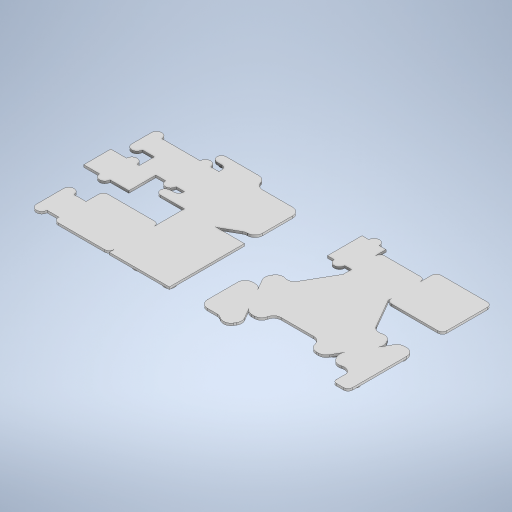
# Autodesk Inventor part: CORE_set_outline
Saved by Autodesk Inventor 2024.1 (Build 281209000, 209)
## iProperties
Created: 2025-04-12
Part Number: CORE_set_outline
Material: 一般
Document SubType Name: Modeling
Designer: hibik
Density: 1 g/cm^3
Appearance: 既定
Author: hibik
Autodesk Inventor part; units mm, degrees
ref_plane "YZ Plane" through (0, 0, 0) normal (1, 0, 0) x (0, 1, 0)
ref_plane "XZ Plane" through (0, 0, 0) normal (0, 1, 0) x (-1, 0, 0)
ref_plane "XY Plane" through (0, 0, 0) normal (0, 0, 1) x (1, 0, 0)
sketch "スケッチ8" plane through (0, 0, 0) normal (0, 1, 0) x (-1, 0, 0)
  line L0 (15, -121.1) -> (15, -99.7075) projected
  arc A0 (15.25, -99.213) -> (15, -99.7075) centre (19.5802, -101.713) ccw projected
  line L1 (15.25, -99.213) -> (26.142, -80.3476) projected
  arc A1 (32.0798, -78.1131) -> (26.142, -80.3476) centre (30.4721, -82.8476) ccw projected
  arc A2 (32.0798, -78.1131) -> (38.0175, -75.8786) centre (33.6874, -73.3786) ccw projected
  line L2 (38.0175, -75.8786) -> (38.7859, -74.5477) projected
  arc A3 (38.7859, -74.5477) -> (38.7859, -69.5477) centre (34.4558, -72.0477) ccw projected
  line L3 (38.7859, -69.5477) -> (26.6628, -48.55) projected
  arc A4 (26.6628, -48.55) -> (22.3327, -46.05) centre (22.3327, -51.05) ccw projected
  line L4 (22.3327, -46.05) -> (20.604, -46.05) projected
  arc A5 (20.604, -46.05) -> (15.7, -50.075) centre (20.604, -51.05) ccw projected
  arc A6 (10.796, -54.1) -> (15.7, -50.075) centre (10.796, -49.1) ccw projected
  line L5 (10.796, -54.1) -> (-10.988, -54.1) projected
  arc A7 (-15.892, -50.075) -> (-10.988, -54.1) centre (-10.988, -49.1) ccw projected
  arc A8 (-15.892, -50.075) -> (-20.796, -46.05) centre (-20.796, -51.05) ccw projected
  line L6 (-20.796, -46.05) -> (-22.3327, -46.05) projected
  arc A9 (-22.3327, -46.05) -> (-26.6628, -48.55) centre (-22.3327, -51.05) ccw projected
  line L7 (-26.6628, -48.55) -> (-38.7859, -69.5477) projected
  arc A10 (-38.7859, -69.5477) -> (-38.7859, -74.5477) centre (-34.4558, -72.0477) ccw projected
  line L8 (-38.7859, -74.5477) -> (-37.9215, -76.0448) projected
  arc A11 (-37.9215, -76.0448) -> (-31.9838, -78.2793) centre (-33.5914, -73.5448) ccw projected
  arc A12 (-26.046, -80.5138) -> (-31.9838, -78.2793) centre (-30.3761, -83.0138) ccw projected
  line L9 (-26.046, -80.5138) -> (-15.154, -99.3793) projected
  arc A13 (-15, -99.6675) -> (-15.154, -99.3793) centre (-19.4842, -101.8793) ccw projected
  line L10 (-15, -99.6675) -> (-15, -121.1) projected
  arc A14 (-15, -121.1) -> (-12, -124.1) centre (-12, -121.1) ccw projected
  line L11 (-12, -124.1) -> (12, -124.1) projected
  arc A15 (12, -124.1) -> (15, -121.1) centre (12, -121.1) ccw projected
  arc A16 (-43.4038, -36.5236) -> (-45.4038, -34.5236) centre (-45.4038, -36.5236) ccw projected
  line L12 (-45.4038, -34.5236) -> (-50.4038, -34.5236) projected
  arc A17 (-50.4038, -34.5236) -> (-53.4038, -37.5236) centre (-50.4038, -37.5236) ccw projected
  line L13 (-53.4038, -37.5236) -> (-53.4038, -73.5448) projected
  arc A18 (-53.4038, -73.5448) -> (-48.4038, -78.5448) centre (-48.4038, -73.5448) ccw projected
  line L14 (-48.4038, -78.5448) -> (-46.8671, -78.5448) projected
  arc A19 (-46.8671, -78.5448) -> (-42.537, -76.0448) centre (-46.8671, -73.5448) ccw projected
  line L15 (-42.537, -76.0448) -> (-30.4139, -55.0471) projected
  arc A20 (-30.4139, -55.0471) -> (-30.4139, -50.0471) centre (-34.7441, -52.5471) ccw projected
  line L16 (-30.4139, -50.0471) -> (-31.2783, -48.55) projected
  arc A21 (-31.2783, -48.55) -> (-37.2161, -46.3155) centre (-35.6084, -51.05) ccw projected
  arc A22 (-43.1538, -44.081) -> (-37.2161, -46.3155) centre (-38.8237, -41.581) ccw projected
  line L17 (-43.1538, -44.081) -> (-43.4038, -43.6479) projected
  line L18 (-43.4038, -43.6479) -> (-43.4038, -36.5236) projected
  arc A23 (-49, -98.6929) -> (-52, -101.6929) centre (-49, -101.6929) ccw projected
  line L19 (-52, -101.6929) -> (-52, -128.6929) projected
  arc A24 (-52, -128.6929) -> (-49, -131.6929) centre (-49, -128.6929) ccw projected
  line L20 (-49, -131.6929) -> (-18, -131.6929) projected
  arc A25 (-18, -131.6929) -> (-15, -128.6929) centre (-18, -128.6929) ccw projected
  line L21 (-15, -128.6929) -> (-15, -101.6929) projected
  arc A26 (-15, -101.6929) -> (-18, -98.6929) centre (-18, -101.6929) ccw projected
  line L22 (-18, -98.6929) -> (-49, -98.6929) projected
  line L23 (26.5, -128.1929) -> (31, -128.1929) projected
  line L24 (31, -128.1929) -> (31, -105.1929) projected
  line L25 (31, -105.1929) -> (26.5, -105.1929) projected
  arc A27 (26.5, -105.1929) -> (19.5, -105.1929) centre (23, -105.1929) ccw projected
  line L26 (19.5, -105.1929) -> (15, -105.1929) projected
  line L27 (15, -105.1929) -> (15, -128.1929) projected
  line L28 (15, -128.1929) -> (19.5, -128.1929) projected
  arc A28 (19.5, -128.1929) -> (26.5, -128.1929) centre (23, -128.1929) ccw projected
  arc A29 (45.5962, -39.8878) -> (40.5962, -34.8878) centre (40.5962, -39.8878) ccw projected
  line L29 (40.5962, -34.8878) -> (34.1859, -34.8878) projected
  arc A30 (31.6859, -34.2179) -> (34.1859, -34.8878) centre (34.1859, -29.8878) ccw projected
  line L30 (31.6859, -34.2179) -> (30.2047, -33.3628) projected
  arc A31 (30.2047, -33.3628) -> (23.3746, -35.1929) centre (27.7047, -37.6929) ccw projected
  line L31 (23.3746, -35.1929) -> (22.6062, -36.5238) projected
  arc A32 (22.6062, -36.5238) -> (22.6062, -41.5238) centre (26.9364, -39.0238) ccw projected
  line L32 (22.6062, -41.5238) -> (34.7293, -62.5215) projected
  arc A33 (34.7293, -62.5215) -> (39.0594, -65.0215) centre (39.0594, -60.0215) ccw projected
  line L33 (39.0594, -65.0215) -> (40.5962, -65.0215) projected
  arc A34 (40.5962, -65.0215) -> (45.5962, -60.0215) centre (40.5962, -60.0215) ccw projected
  line L34 (45.5962, -60.0215) -> (45.5962, -39.8878) projected
  arc A35 (70.5962, -91.5196) -> (65.5962, -96.5196) centre (70.5962, -96.5196) ccw projected
  line L35 (65.5962, -96.5196) -> (65.5962, -116.5196) projected
  arc A36 (65.5962, -116.5196) -> (70.5962, -121.5196) centre (70.5962, -116.5196) ccw projected
  line L36 (70.5962, -121.5196) -> (90.5124, -121.5196) projected
  arc A37 (95.2815, -125.0175) -> (90.5124, -121.5196) centre (90.5124, -126.5196) ccw projected
  arc A38 (95.2815, -125.0175) -> (100.0506, -128.5155) centre (100.0506, -123.5155) ccw projected
  line L37 (100.0506, -128.5155) -> (121.8354, -128.5155) projected
  arc A39 (121.8354, -128.5155) -> (123.6192, -123.1035) centre (121.8354, -125.5155) ccw projected
  arc A40 (123.6192, -123.1035) -> (122.0183, -122.3155) centre (120.6462, -127.1236) ccw projected
  line L38 (122.0183, -122.3155) -> (118.5962, -122.3155) projected
  arc A41 (115.5962, -119.3155) -> (118.5962, -122.3155) centre (118.5962, -119.3155) ccw projected
  line L39 (115.5962, -119.3155) -> (115.5962, -93.7236) projected
  arc A42 (118.5962, -90.7236) -> (115.5962, -93.7236) centre (118.5962, -93.7236) ccw projected
  line L40 (118.5962, -90.7236) -> (121.224, -90.7236) projected
  arc A43 (121.6212, -90.6276) -> (121.224, -90.7236) centre (122.5962, -95.5316) ccw projected
  arc A44 (121.6212, -90.6276) -> (122.8256, -90.2236) centre (120.6462, -85.7236) ccw projected
  arc A45 (122.8256, -90.2236) -> (121.5179, -84.5236) centre (121.5179, -87.5236) ccw projected
  line L41 (121.5179, -84.5236) -> (84.9713, -84.5236) projected
  arc A46 (84.9713, -84.5236) -> (83.4713, -84.9255) centre (84.9713, -87.5236) ccw projected
  line L42 (83.4713, -84.9255) -> (73.2103, -90.8497) projected
  arc A47 (70.7103, -91.5196) -> (73.2103, -90.8497) centre (70.7103, -86.5196) ccw projected
  line L43 (70.7103, -91.5196) -> (70.5962, -91.5196) projected
  line L44 (121.0962, -94.5155) -> (115.5962, -94.5155) projected
  line L45 (115.5962, -94.5155) -> (115.5962, -117.5155) projected
  line L46 (115.5962, -117.5155) -> (121.0962, -117.5155) projected
  arc A48 (121.0962, -117.5155) -> (128.0962, -117.5155) centre (124.5962, -117.5155) ccw projected
  line L47 (128.0962, -117.5155) -> (145.5962, -117.5155) projected
  line L48 (145.5962, -117.5155) -> (145.5962, -94.5155) projected
  line L49 (145.5962, -94.5155) -> (128.0962, -94.5155) projected
  arc A49 (128.0962, -94.5155) -> (121.0962, -94.5155) centre (124.5962, -94.5155) ccw projected
  line L50 (153.5962, -104.5155) -> (145.5962, -104.5155) projected
  line L51 (145.5962, -104.5155) -> (145.5962, -117.5155) projected
  line L52 (145.5962, -117.5155) -> (153.5962, -117.5155) projected
  arc A50 (153.5962, -117.5155) -> (160.5962, -117.5155) centre (157.0962, -117.5155) ccw projected
  line L53 (160.5962, -117.5155) -> (160.5962, -104.5155) projected
  arc A51 (160.5962, -104.5155) -> (153.5962, -104.5155) centre (157.0962, -104.5155) ccw projected
  line L54 (147.0962, -76.5155) -> (134.5962, -76.5155) projected
  line L55 (134.5962, -76.5155) -> (134.5962, -94.5155) projected
  line L56 (134.5962, -94.5155) -> (147.0962, -94.5155) projected
  arc A52 (147.0962, -94.5155) -> (154.0962, -94.5155) centre (150.5962, -94.5155) ccw projected
  line L57 (154.0962, -94.5155) -> (164.5962, -94.5155) projected
  line L58 (164.5962, -94.5155) -> (164.5962, -76.5155) projected
  line L59 (164.5962, -76.5155) -> (154.0962, -76.5155) projected
  arc A53 (154.0962, -76.5155) -> (147.0962, -76.5155) centre (150.5962, -76.5155) ccw projected
  line L60 (65.5962, -84.5236) -> (105.5962, -84.5236) projected
  line L61 (105.5962, -84.5236) -> (105.5962, -54.5236) projected
  line L62 (105.5962, -54.5236) -> (65.5962, -54.5236) projected
  line L63 (65.5962, -54.5236) -> (65.5962, -84.5236) projected
  line L64 (65.5962, -54.5236) -> (105.5962, -54.5236) projected
  line L65 (105.5962, -54.5236) -> (105.5962, -34.5236) projected
  line L66 (105.5962, -34.5236) -> (65.5962, -34.5236) projected
  line L67 (65.5962, -34.5236) -> (65.5962, -54.5236) projected
  arc A54 (108.5962, -34.5236) -> (105.5962, -37.5236) centre (108.5962, -37.5236) ccw projected
  line L68 (105.5962, -37.5236) -> (105.5962, -64.5236) projected
  arc A55 (105.5962, -64.5236) -> (108.5962, -67.5236) centre (108.5962, -64.5236) ccw projected
  line L69 (108.5962, -67.5236) -> (139.5962, -67.5236) projected
  arc A56 (139.5962, -67.5236) -> (142.5962, -64.5236) centre (139.5962, -64.5236) ccw projected
  line L70 (142.5962, -64.5236) -> (142.5962, -37.5236) projected
  arc A57 (142.5962, -37.5236) -> (139.5962, -34.5236) centre (139.5962, -37.5236) ccw projected
  line L71 (139.5962, -34.5236) -> (108.5962, -34.5236) projected
  line L72 (157.5962, -56.0236) -> (157.5962, -38.0236) projected
  arc A58 (157.5962, -38.0236) -> (150.5962, -38.0236) centre (154.0962, -38.0236) ccw projected
  line L73 (150.5962, -38.0236) -> (142.5962, -38.0236) projected
  line L74 (142.5962, -38.0236) -> (142.5962, -56.0236) projected
  line L75 (142.5962, -56.0236) -> (150.5962, -56.0236) projected
  arc A59 (150.5962, -56.0236) -> (157.5962, -56.0236) centre (154.0962, -56.0236) ccw projected
  point P0 (0, 0)
extrude "押し出し6" add sketch "スケッチ8" along normal blind 1.5
sketch "スケッチ9" plane through (0, 1.5, 0) normal (0, 1, 0) x (1, 0, 0)
  line L0 (-22.6062, 41.5238) -> (-26.6628, 48.55) projected
  arc A0 (-26.6628, 48.55) -> (-22.3327, 46.05) centre (-22.3327, 51.05) ccw projected
  line L1 (-22.3327, 46.05) -> (-20.604, 46.05) projected
  arc A1 (-20.604, 46.05) -> (-15.7, 50.075) centre (-20.604, 51.05) ccw projected
  arc A2 (-10.796, 54.1) -> (-15.7, 50.075) centre (-10.796, 49.1) ccw projected
  line L2 (-10.796, 54.1) -> (10.988, 54.1) projected
  arc A3 (15.892, 50.075) -> (10.988, 54.1) centre (10.988, 49.1) ccw projected
  arc A4 (15.892, 50.075) -> (20.796, 46.05) centre (20.796, 51.05) ccw projected
  line L3 (20.796, 46.05) -> (22.3327, 46.05) projected
  arc A5 (22.3327, 46.05) -> (26.6628, 48.55) centre (22.3327, 51.05) ccw projected
  line L4 (26.6628, 48.55) -> (30.4139, 55.0471) projected
  arc A6 (30.4139, 55.0471) -> (30.4139, 50.0471) centre (34.7441, 52.5471) ccw projected
  line L5 (30.4139, 50.0471) -> (31.2783, 48.55) projected
  arc A7 (31.2783, 48.55) -> (37.2161, 46.3155) centre (35.6084, 51.05) ccw projected
  arc A8 (43.1538, 44.081) -> (37.2161, 46.3155) centre (38.8237, 41.581) ccw projected
  line L6 (43.1538, 44.081) -> (43.4038, 43.6479) projected
  line L7 (43.4038, 43.6479) -> (43.4038, 36.5236) projected
  arc A9 (43.4038, 36.5236) -> (45.4038, 34.5236) centre (45.4038, 36.5236) ccw projected
  line L8 (45.4038, 34.5236) -> (50.4038, 34.5236) projected
  arc A10 (50.4038, 34.5236) -> (53.4038, 37.5236) centre (50.4038, 37.5236) ccw projected
  line L9 (53.4038, 37.5236) -> (53.4038, 73.5448) projected
  arc A11 (53.4038, 73.5448) -> (48.4038, 78.5448) centre (48.4038, 73.5448) ccw projected
  line L10 (48.4038, 78.5448) -> (46.8671, 78.5448) projected
  arc A12 (46.8671, 78.5448) -> (42.537, 76.0448) centre (46.8671, 73.5448) ccw projected
  line L11 (42.537, 76.0448) -> (38.7859, 69.5477) projected
  arc A13 (38.7859, 69.5477) -> (38.7859, 74.5477) centre (34.4558, 72.0477) ccw projected
  line L12 (38.7859, 74.5477) -> (37.9215, 76.0448) projected
  arc A14 (37.9215, 76.0448) -> (31.9838, 78.2793) centre (33.5914, 73.5448) ccw projected
  arc A15 (26.046, 80.5138) -> (31.9838, 78.2793) centre (30.3761, 83.0138) ccw projected
  line L13 (26.046, 80.5138) -> (15.154, 99.3793) projected
  arc A16 (15, 99.6675) -> (15.154, 99.3793) centre (19.4842, 101.8793) ccw projected
  line L14 (15, 99.6675) -> (15, 101.6929) projected
  arc A17 (15, 101.6929) -> (18, 98.6929) centre (18, 101.6929) ccw projected
  line L15 (18, 98.6929) -> (49, 98.6929) projected
  arc A18 (49, 98.6929) -> (52, 101.6929) centre (49, 101.6929) ccw projected
  line L16 (52, 101.6929) -> (52, 128.6929) projected
  arc A19 (52, 128.6929) -> (49, 131.6929) centre (49, 128.6929) ccw projected
  line L17 (49, 131.6929) -> (18, 131.6929) projected
  arc A20 (18, 131.6929) -> (15, 128.6929) centre (18, 128.6929) ccw projected
  line L18 (15, 128.6929) -> (15, 121.1) projected
  arc A21 (15, 121.1) -> (12, 124.1) centre (12, 121.1) ccw projected
  line L19 (12, 124.1) -> (-12, 124.1) projected
  arc A22 (-12, 124.1) -> (-15, 121.1) centre (-12, 121.1) ccw projected
  line L20 (-15, 121.1) -> (-15, 128.1929) projected
  line L21 (-15, 128.1929) -> (-19.5, 128.1929) projected
  arc A23 (-19.5, 128.1929) -> (-26.5, 128.1929) centre (-23, 128.1929) ccw projected
  line L22 (-26.5, 128.1929) -> (-31, 128.1929) projected
  line L23 (-31, 128.1929) -> (-31, 105.1929) projected
  line L24 (-31, 105.1929) -> (-26.5, 105.1929) projected
  arc A24 (-26.5, 105.1929) -> (-19.5, 105.1929) centre (-23, 105.1929) ccw projected
  line L25 (-19.5, 105.1929) -> (-15, 105.1929) projected
  line L26 (-15, 105.1929) -> (-15, 99.7075) projected
  arc A25 (-15.25, 99.213) -> (-15, 99.7075) centre (-19.5802, 101.713) ccw projected
  line L27 (-15.25, 99.213) -> (-26.142, 80.3476) projected
  arc A26 (-32.0798, 78.1131) -> (-26.142, 80.3476) centre (-30.4721, 82.8476) ccw projected
  arc A27 (-32.0798, 78.1131) -> (-38.0175, 75.8786) centre (-33.6874, 73.3786) ccw projected
  line L28 (-38.0175, 75.8786) -> (-38.7859, 74.5477) projected
  arc A28 (-38.7859, 74.5477) -> (-38.7859, 69.5477) centre (-34.4558, 72.0477) ccw projected
  line L29 (-38.7859, 69.5477) -> (-34.7293, 62.5215) projected
  arc A29 (-34.7293, 62.5215) -> (-39.0594, 65.0215) centre (-39.0594, 60.0215) ccw projected
  line L30 (-39.0594, 65.0215) -> (-40.5962, 65.0215) projected
  arc A30 (-40.5962, 65.0215) -> (-45.5962, 60.0215) centre (-40.5962, 60.0215) ccw projected
  line L31 (-45.5962, 60.0215) -> (-45.5962, 39.8878) projected
  arc A31 (-45.5962, 39.8878) -> (-40.5962, 34.8878) centre (-40.5962, 39.8878) ccw projected
  line L32 (-40.5962, 34.8878) -> (-34.1859, 34.8878) projected
  arc A32 (-31.6859, 34.2179) -> (-34.1859, 34.8878) centre (-34.1859, 29.8878) ccw projected
  line L33 (-31.6859, 34.2179) -> (-30.2047, 33.3628) projected
  arc A33 (-30.2047, 33.3628) -> (-23.3746, 35.1929) centre (-27.7047, 37.6929) ccw projected
  line L34 (-23.3746, 35.1929) -> (-22.6062, 36.5238) projected
  arc A34 (-22.6062, 36.5238) -> (-22.6062, 41.5238) centre (-26.9364, 39.0238) ccw projected
  line L35 (-65.5962, 84.5236) -> (-84.9713, 84.5236) projected
  arc A35 (-84.9713, 84.5236) -> (-83.4713, 84.9255) centre (-84.9713, 87.5236) ccw projected
  line L36 (-83.4713, 84.9255) -> (-73.2103, 90.8497) projected
  arc A36 (-70.7103, 91.5196) -> (-73.2103, 90.8497) centre (-70.7103, 86.5196) ccw projected
  line L37 (-70.7103, 91.5196) -> (-70.5962, 91.5196) projected
  arc A37 (-70.5962, 91.5196) -> (-65.5962, 96.5196) centre (-70.5962, 96.5196) ccw projected
  line L38 (-65.5962, 96.5196) -> (-65.5962, 116.5196) projected
  arc A38 (-65.5962, 116.5196) -> (-70.5962, 121.5196) centre (-70.5962, 116.5196) ccw projected
  line L39 (-70.5962, 121.5196) -> (-90.5124, 121.5196) projected
  arc A39 (-95.2815, 125.0175) -> (-90.5124, 121.5196) centre (-90.5124, 126.5196) ccw projected
  arc A40 (-95.2815, 125.0175) -> (-100.0506, 128.5155) centre (-100.0506, 123.5155) ccw projected
  line L40 (-100.0506, 128.5155) -> (-121.8354, 128.5155) projected
  arc A41 (-121.8354, 128.5155) -> (-123.6192, 123.1035) centre (-121.8354, 125.5155) ccw projected
  arc A42 (-123.6192, 123.1035) -> (-122.0183, 122.3155) centre (-120.6462, 127.1236) ccw projected
  line L41 (-122.0183, 122.3155) -> (-118.5962, 122.3155) projected
  arc A43 (-115.5962, 119.3155) -> (-118.5962, 122.3155) centre (-118.5962, 119.3155) ccw projected
  line L42 (-115.5962, 119.3155) -> (-115.5962, 117.5155) projected
  line L43 (-115.5962, 117.5155) -> (-121.0962, 117.5155) projected
  arc A44 (-121.0962, 117.5155) -> (-128.0962, 117.5155) centre (-124.5962, 117.5155) ccw projected
  line L44 (-128.0962, 117.5155) -> (-153.5962, 117.5155) projected
  arc A45 (-153.5962, 117.5155) -> (-160.5962, 117.5155) centre (-157.0962, 117.5155) ccw projected
  line L45 (-160.5962, 117.5155) -> (-160.5962, 104.5155) projected
  arc A46 (-160.5962, 104.5155) -> (-153.5962, 104.5155) centre (-157.0962, 104.5155) ccw projected
  line L46 (-153.5962, 104.5155) -> (-145.5962, 104.5155) projected
  line L47 (-145.5962, 104.5155) -> (-145.5962, 94.5155) projected
  line L48 (-145.5962, 94.5155) -> (-147.0962, 94.5155) projected
  arc A47 (-147.0962, 94.5155) -> (-154.0962, 94.5155) centre (-150.5962, 94.5155) ccw projected
  line L49 (-154.0962, 94.5155) -> (-164.5962, 94.5155) projected
  line L50 (-164.5962, 94.5155) -> (-164.5962, 76.5155) projected
  line L51 (-164.5962, 76.5155) -> (-154.0962, 76.5155) projected
  arc A48 (-154.0962, 76.5155) -> (-147.0962, 76.5155) centre (-150.5962, 76.5155) ccw projected
  line L52 (-147.0962, 76.5155) -> (-134.5962, 76.5155) projected
  line L53 (-134.5962, 76.5155) -> (-134.5962, 94.5155) projected
  line L54 (-134.5962, 94.5155) -> (-128.0962, 94.5155) projected
  arc A49 (-128.0962, 94.5155) -> (-121.0962, 94.5155) centre (-124.5962, 94.5155) ccw projected
  line L55 (-121.0962, 94.5155) -> (-115.5962, 94.5155) projected
  line L56 (-115.5962, 94.5155) -> (-115.5962, 93.7236) projected
  arc A50 (-118.5962, 90.7236) -> (-115.5962, 93.7236) centre (-118.5962, 93.7236) ccw projected
  line L57 (-118.5962, 90.7236) -> (-121.224, 90.7236) projected
  arc A51 (-121.6212, 90.6276) -> (-121.224, 90.7236) centre (-122.5962, 95.5316) ccw projected
  arc A52 (-121.6212, 90.6276) -> (-122.8256, 90.2236) centre (-120.6462, 85.7236) ccw projected
  arc A53 (-122.8256, 90.2236) -> (-121.5179, 84.5236) centre (-121.5179, 87.5236) ccw projected
  line L58 (-121.5179, 84.5236) -> (-105.5962, 84.5236) projected
  line L59 (-105.5962, 84.5236) -> (-105.5962, 64.5236) projected
  arc A54 (-105.5962, 64.5236) -> (-108.5962, 67.5236) centre (-108.5962, 64.5236) ccw projected
  line L60 (-108.5962, 67.5236) -> (-139.5962, 67.5236) projected
  arc A55 (-139.5962, 67.5236) -> (-142.5962, 64.5236) centre (-139.5962, 64.5236) ccw projected
  line L61 (-142.5962, 64.5236) -> (-142.5962, 56.0236) projected
  line L62 (-142.5962, 56.0236) -> (-150.5962, 56.0236) projected
  arc A56 (-150.5962, 56.0236) -> (-157.5962, 56.0236) centre (-154.0962, 56.0236) ccw projected
  line L63 (-157.5962, 56.0236) -> (-157.5962, 38.0236) projected
  arc A57 (-157.5962, 38.0236) -> (-150.5962, 38.0236) centre (-154.0962, 38.0236) ccw projected
  line L64 (-150.5962, 38.0236) -> (-142.5962, 38.0236) projected
  line L65 (-142.5962, 38.0236) -> (-142.5962, 37.5236) projected
  arc A58 (-142.5962, 37.5236) -> (-139.5962, 34.5236) centre (-139.5962, 37.5236) ccw projected
  line L66 (-139.5962, 34.5236) -> (-108.5962, 34.5236) projected
  arc A59 (-108.5962, 34.5236) -> (-105.5962, 37.5236) centre (-108.5962, 37.5236) ccw projected
  line L67 (-105.5962, 37.5236) -> (-105.5962, 34.5236) projected
  line L68 (-105.5962, 34.5236) -> (-65.5962, 34.5236) projected
  line L69 (-65.5962, 34.5236) -> (-65.5962, 84.5236) projected
  circle A60 centre (51.4038, 41.8946) radius 2
  circle A61 centre (51.4038, 72.5448) radius 2
  circle A62 centre (42.8257, 72.5448) radius 2
  circle A63 centre (26.3742, 52.05) radius 2
  circle A64 centre (-26.403, 52.1) radius 2
  circle A65 centre (-35.018, 59.0215) radius 2
  circle A66 centre (-43.5962, 59.0215) radius 2
  circle A67 centre (-18.964, 88.7803) radius 2
  circle A68 centre (10.2802, 83.821) radius 2
  circle A69 centre (0.096, 66.1) radius 2
  circle A70 centre (0.096, 77.776) radius 2
  circle A71 centre (-11.5, 62.6) radius 1.5
  circle A72 centre (11.5, 62.6) radius 1.5
  circle A73 centre (11.5, 120.6) radius 1.5
  circle A74 centre (-23, 105.1929) radius 2
  circle A75 centre (-23, 128.1929) radius 2
  circle A76 centre (-23, 116.6929) radius 2
  circle A77 centre (-119.6462, 124.3155) radius 2
  circle A78 centre (-119.6462, 88.7236) radius 2
  circle A79 centre (-124.5962, 94.5155) radius 2
  circle A80 centre (-124.5962, 117.5155) radius 2
  circle A81 centre (-124.5962, 106.0155) radius 2
  circle A82 centre (-157.0962, 104.5155) radius 2
  circle A83 centre (-157.0962, 117.5155) radius 2
  circle A84 centre (-147.5962, 111.0155) radius 2
  circle A85 centre (-150.5962, 76.5155) radius 2
  circle A86 centre (-150.5962, 94.5155) radius 2
  circle A87 centre (-150.5962, 85.5155) radius 2
  circle A88 centre (-154.0962, 38.0236) radius 2
  circle A89 centre (-154.0962, 56.0236) radius 2
  circle A90 centre (-144.5962, 47.0236) radius 2
  circle A91 centre (-69.0962, 38.0236) radius 3.5
  circle A92 centre (-89.0962, 38.0236) radius 3.5
  circle A93 centre (-83.5962, 58.0236) radius 3.5
  circle A94 centre (-83.5962, 81.0236) radius 3.5
  circle A95 centre (-94.0962, 69.5236) radius 2
  line L70 (-89.5962, 63.5236) -> (-98.5962, 63.5236)
  line L71 (-98.5962, 63.5236) -> (-98.5962, 75.5236)
  line L72 (-98.5962, 75.5236) -> (-89.5962, 75.5236)
  line L73 (-89.5962, 75.5236) -> (-89.5962, 63.5236)
  line L74 (-65.5962, 84.5236) -> (-105.5962, 84.5236)
  line L75 (-105.5962, 84.5236) -> (-105.5962, 54.5236)
  line L76 (-105.5962, 54.5236) -> (-65.5962, 54.5236)
  line L77 (-65.5962, 54.5236) -> (-65.5962, 84.5236)
  line L78 (-105.5962, 84.5236) -> (-105.5962, 64.5236) projected
  line L79 (0, 158.7771) -> (0, -26.4628) construction
  line L80 (0.096, 54.1) -> (0.096, 77.776) construction
  line L81 (-10.796, 54.1) -> (10.988, 54.1) projected
  line L82 (0.096, 77.776) -> (20.6, 89.9466) construction
  line L83 (0.096, 77.776) -> (-20.696, 89.7803) construction
  line L84 (-15.25, 99.213) -> (-26.142, 80.3476) projected
  line L85 (26.6628, 48.55) -> (30.4139, 55.0471) projected
  line L86 (-22.6062, 41.5238) -> (-26.6628, 48.55) projected
  line L87 (42.537, 76.0448) -> (38.7859, 69.5477) projected
  line L88 (53.4038, 37.5236) -> (53.4038, 73.5448) projected
  line L89 (-38.7859, 69.5477) -> (-34.7293, 62.5215) projected
  line L90 (-45.5962, 60.0215) -> (-45.5962, 39.8878) projected
  line L91 (-142.5962, 64.5236) -> (-142.5962, 56.0236) projected
  line L92 (-118.5962, 90.7236) -> (-121.224, 90.7236) projected
  line L93 (-105.5962, 34.5236) -> (-65.5962, 34.5236) projected
  line L94 (-65.5962, 34.5236) -> (-65.5962, 84.5236) projected
  circle A96 centre (-89.9201, 106.0155) radius 2
  point P0 (0, 0)
  point P1 (-98.5962, 69.5236)
  point P2 (-105.5962, 69.5236)
  point P3 (-94.0962, 63.5236)
  point P4 (-31, 116.6929)
  point P5 (-160.5962, 111.0155)
  point P6 (-164.5962, 85.5155)
  point P7 (-157.5962, 47.0236)
  dimension "d12" = 30
  dimension "d13" = 7
  dimension "d14" = 9
  dimension "d15" = 12
  dimension "d16" = 7
  dimension "d17" = 4
  dimension "d18" = 3
  dimension "d19" = 23
  dimension "d20" = 58
  dimension "d21" = 3.5
  dimension "d22" = 12
  dimension "d23" = 12
  dimension "d24" = 6
  dimension "d25" = 6
  dimension "d26" = 6
  dimension "d27" = 4.371
  dimension "d28" = 18
  dimension "d29" = 11.5
  dimension "d30" = 11.5
  dimension "d31" = 4.05
  dimension "d32" = 20
  dimension "d35" = 23.676
  dimension "d36" = 11.5
  dimension "d37" = 11.5
  dimension "d38" = 25.676
  constraints: 37 centre point, 34 equal radius, 22 end point, 18 tangent, 10 coincident, 10 midpoint, 9 horizontal alignment, 8 vertical alignment, 4 parallel, 4 perpendicular, 2 horizontal, 2 point on line, 1 collinear, 1 symmetric about line
  measures "d12" distance of L74.end L75.end
  measures "d13" diameter of A91
  measures "d14" distance of L71.end L72.end
  measures "d15" distance of L70.end L71.end
  measures "d16" distance between parallel lines of L75 L71
  measures "d17" diameter of A70
  measures "d18" diameter of A72
  measures "d19" distance of A71.centre A72.centre
  measures "d20" distance of A73.centre A72.centre
  measures "d21" distance from line of L19 A73.centre
  measures "d22" distance from line of L2 A69.centre
  measures "d23" distance from line of L13 A68.centre
  measures "d24" distance from line of L3 A63.centre
  measures "d25" distance from line of L30 A65.centre
  measures "d26" distance from line of L10 A62.centre
  measures "d27" vertical distance of A10.centre A60.centre
  measures "d28" distance from line of L69 A93.centre
  measures "d29" distance of A49.centre A81.centre
  measures "d30" distance of A44.centre A81.centre
  measures "d31" horizontal distance of A78.centre L55.end
  measures "d32" distance of A92.centre A91.centre
  measures "d35" distance from line of L80.end L2
  measures "d36" distance from line of L43 A96.centre
  measures "d37" distance from line of A96.centre L55
  measures "d38" horizontal distance of L42.end A96.centre
extrude "押し出し7" add sketch "スケッチ9" against normal blind 2 contours A63 | A60 | A61 | A62 | A67 | A66 | A94 | A93 | A92 | A77 | A78 | A91 | A64 | A65 | A68 | A69 | A70 | A71 | A72 | A73 | A74 | A75 | A76 | A79 | A80 | A81 | A82 | A83 | A84 | A85 | A86 | A87 | A88 | A89 | A90 | A95 | A96
equation "\"d23\" = d22"
equation "\"d25\" = d24"
equation "\"d26\" = d24"
equation "\"d29\" = d30"
equation "\"d36\" = d37"
